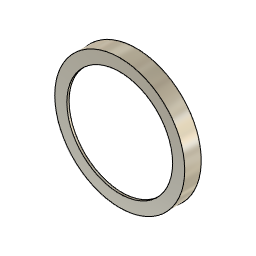
灯 v4 v2 (Autodesk Fusion 360 design; units mm, degrees)
Autodesk Fusion 360 part; units mm, degrees
note: some values were not read from the file. Set by a fixed rule: which sketch regions a step uses.
sketch "草图1" plane through (0, 0, 0) normal (0, 1, 0) x (1, 0, 0)
  circle A0 centre (0, 0) radius 29.5
  line L0 (0, 0) -> (0, 29.5) construction
  dimension "d1" = 59
  constraint coincident A0.centre L0.start
  constraint coincident A0 L0.end
  constraint vertical L0
  measures "d1" diameter of A0
extrude "拉伸1" add sketch "草图1" along normal blind 7.5
sketch "草图2" plane through (0, 0, 0) normal (0, -1, 0) x (1, 0, 0)
  circle A0 centre (0, 0) radius 29.5
  circle A1 centre (0, 0) radius 24
  dimension "d5" = 48
  dimension "d6" = 48
  constraint concentric A0 A1
  measures "d5" diameter of A1
  measures "d6" diameter of A1
extrude "拉伸2" cut sketch "草图2" against normal blind 1 contours A1
sketch "草图3" plane through (0, 7.5, 0) normal (0, 1, 0) x (-1, 0, 0)
  circle A0 centre (0, 0) radius 29.5
  line L0 (-2, -23.4321) -> (-2, -29.4321)
  line L1 (2, -23.4321) -> (2, -29.4321)
  line L2 (0, 0) -> (0, -21.4321) construction
  arc A1 (2, -23.4321) -> (-2, -23.4321) centre (0, -23.4321) ccw
  dimension "d9" = 6
  dimension "d10" = 2
  dimension "d11" = 6
  dimension "d12" = 2
  dimension "d13" = 2
  constraint coincident A0.centre L2.start
  constraint vertical L2
  constraint coincident A0 L0.end
  constraint vertical L0
  constraint coincident A0 L1.end
  constraint parallel L1 L2
  constraint coincident A1.centre L2
  constraint coincident L2.end A1
  measures "d9" distance of L0.start L0.end
  measures "d10" distance of L0 L2
  measures "d11" distance of L1.start L1.end
  measures "d12" distance of L1 L2
  measures "d13" radius of A1
extrude "拉伸3" cut sketch "草图3" against normal blind 2 contours A0 L0 L1 A1 picked at (0.2224, -25.4522)
